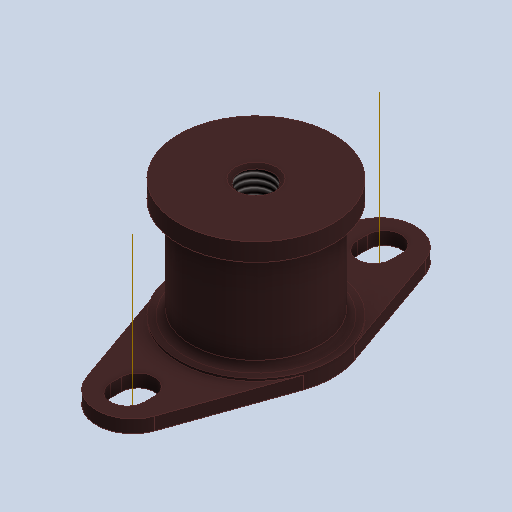
# Autodesk Inventor part: NHF19-3026-M8
Saved by Autodesk Inventor 2025.2 (Build 292293000, 293)
## iProperties
Category: PARTsolutions
Company: YIHEDA
Created: 2025-06-22
Part Number: NHF19-3026-M8
Material: Generic
Catalog Web Link: www.cadenas.de
Description: NHF19-Rubber shock absorber, internal thread fixing plate
Vendor: YIHEDA
Document SubType Name: Modeling
Designer: psAdmin
Manufacturer: YIHEDA
Mass: 14.9467 g
Surface Area: 53.4793 cm^2
Volume: 14.9467 cm^3
Density: 1 g/cm^3
Appearance: PSOLRGB-175-175-175
PSOL_IDENT_0: {$CADENAS_DATA/23d-libs/yiheda/yhd_fa/g3/nhf19.prj},166 {VTYP=3D},{NB=NHF19-3026-M8},{LINA=NHF19-302
PSOL_IDENT_1: 6-M8},{NN=NHF19},{DATE=08.04.2025 03:07:34},{GEOMDATE=19.08.2021 06:01:30},{VERSION=},{LINEID=440},{
PSOL_IDENT_2: WBVAR=},{WBNUMERIC=}  {NB=NHF19-3026-M8},{LINA=NHF19-3026-M8},{KT=DUMMY},{NENN=NHF19-3026-M8},{CODE=
PSOL_IDENT_3: NHF19},{TYPE=Internal thread fixing plate, economical, waist type},{MAT1=natural rubber},{MAT2=S45C}
PSOL_IDENT_4: ,{HRD=Shore A60},{SUR=Galvanized},{SP=3026},{M=8},{D1=30},{D2=25},{H1=26},{H2=20.0},{TT=3.5},{TT1=2.
PSOL_IDENT_5: 5},{L2=8},{W1=62},{W2=30},{E=8.5},{F=6.5},{P=48},{R=7.0},{ZR=760(77)},{ZB=196-370(20-38)},{ZT=180(18
PSOL_IDENT_6: 0)},{XR=150(15)},{RI=0.22},{CNSTYPECODE=NHF19-3026-M8},{LINK=webxxx},{WEB=https://www.yhdfa.com/prod
PSOL_IDENT_7: uct/G/G03_04/NHF19-NHE44?productModel=NHF19-3026-M8}
NB: NHF19-3026-M8
NN: NHF19
NT: Rubber shock absorber, internal thread fixing plate
NBSYN: $NENN.
LINA: NHF19-3026-M8
CATALOG: YIHEDA
ROWDESC: NHF19-3026-M8
CODE: NHF19
TYPE: Internal thread fixing plate, economical, waist type
MAT1: natural rubber
MAT2: S45C
HRD: Shore A60
SUR: Galvanized
SP: 3026
M: 8
D1: 30
D2: 25
H1: 26
H2: 20
TT: 3.5
TT1: 2.5
L2: 8
W1: 62
W2: 30
E: 8.5
F: 6.5
P: 48
ZR: 760(77)
ZB: 196-370(20-38)
ZT: 180(180)
XR: 150(15)
RI: 0.22
LINK: Website connection
SUPPLIER: YIHEDA
ARTICLENO: NHF19-3026-M8
BOMINFO: NHF19-3026-M8
CREATOR: CADENAS GmbH
Title: NHF19-3026-M8
Author: Cadenas PARTsolutions
Comments: Rubber shock absorber, internal thread fixing plate
Autodesk Inventor part; units mm, degrees
ref_plane "XZ Plane" through (0, 0, 0) normal (0, 1, 0) x (-1, 0, 0)
sketch "__1" plane through (0, 0, 0) normal (0, 1, 0) x (-1, 0, 0)
  arc A0 (14.1421, -5) -> (14.1421, 5) centre (0, 0) ccw
  line L0 (14.1421, 5) -> (6.5997, 26.3333)
  arc A1 (6.5997, 26.3333) -> (-6.5997, 26.3333) centre (0, 24) ccw
  line L1 (-6.5997, 26.3333) -> (-14.1421, 5)
  arc A2 (-14.1421, 5) -> (-14.1421, -5) centre (0, 0) ccw
  line L2 (-14.1421, -5) -> (-6.5997, -26.3333)
  arc A3 (-6.5997, -26.3333) -> (6.5997, -26.3333) centre (0, -24) ccw
  line L3 (6.5997, -26.3333) -> (14.1421, -5)
  arc A4 (3.25, -23) -> (-3.25, -23) centre (0, -23) ccw
  line L4 (-3.25, -23) -> (-3.25, -25)
  arc A5 (-3.25, -25) -> (3.25, -25) centre (0, -25) ccw
  line L5 (3.25, -25) -> (3.25, -23)
  line L6 (3.25, 23) -> (3.25, 25)
  arc A6 (3.25, 25) -> (-3.25, 25) centre (0, 25) ccw
  line L7 (-3.25, 25) -> (-3.25, 23)
  arc A7 (-3.25, 23) -> (3.25, 23) centre (0, 23) ccw
  constraints: 16 end point, 16 point on circle, 8 centre point
extrude "Extrusion1" add sketch "__1" along normal blind 2.5
sketch "__2" plane through (0, 0, 0) normal (0, 0, 1) x (1, 0, 0)
  line L0 (0, 2.5) -> (0, 26)
  line L1 (0, 11.9406) -> (3.3235, 13.8594)
  line L2 (3.3235, 13.8594) -> (3.3235, 25.3235)
  line L3 (3.3235, 25.3235) -> (4, 26)
  line L4 (4, 26) -> (15, 26)
  line L5 (15, 26) -> (15, 22.5)
  line L6 (15, 22.5) -> (13.75, 22.5)
  arc A0 (13.75, 22.5) -> (12.5, 21.25) centre (13.75, 21.25) ccw
  line L7 (12.5, 21.25) -> (12.5, 4.25)
  arc A1 (12.5, 4.25) -> (13.75, 3) centre (13.75, 4.25) ccw
  line L8 (13.75, 3) -> (15, 3)
  line L9 (15, 3) -> (15, 2.5)
  line L10 (15, 2.5) -> (0, 2.5)
  line L11 (0, 2.5) -> (0, 11.9406)
  constraints: 24 end point, 4 point on circle, 2 centre point
revolve "Revolution1" add sketch "__2" angle 360 about axis through (0, 2.5, 0) along (0, -1, 0)
thread "Thread1" size "M8x1.25" class "6H" standard "ISO Metric profile" length 7.3235
ref_plane "Arbeitsebene1" through (0, 0, 24) normal (0, 0, 1) x (1, 0, 0)
ref_plane "Arbeitsebene2" through (0, 0, -24) normal (0, 0, 1) x (1, 0, 0)
body "Solid1"
